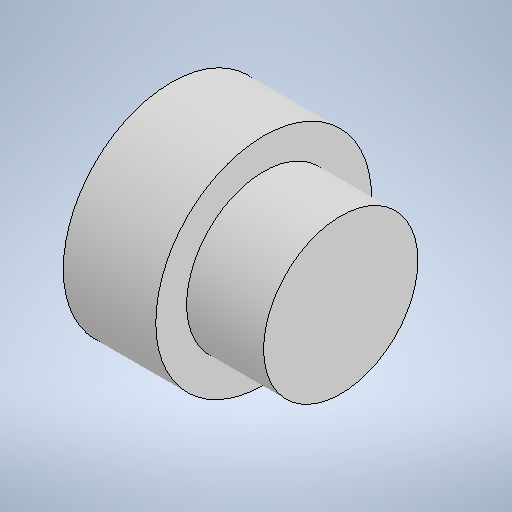
# Autodesk Inventor part: 1 part 16
Saved by Autodesk Inventor 2025 (Build 290162010, 162A)
## iProperties
Created: 2024-07-30
Part Number: 1 part 16
Material: Generic
Document SubType Name: Modeling
Designer: Fabri
Density: 1 g/cm^3
Appearance: Default
Author: Fabri
Autodesk Inventor part; units mm, degrees
ref_plane "YZ Plane" through (0, 0, 0) normal (1, 0, 0) x (0, 1, 0)
ref_plane "XZ Plane" through (0, 0, 0) normal (0, 1, 0) x (-1, 0, 0)
ref_plane "XY Plane" through (0, 0, 0) normal (0, 0, 1) x (1, 0, 0)
sketch "Sketch1" plane through (0, 0, 0) normal (0, 0, 1) x (1, 0, 0)
  line L0 (0, 0) -> (0, 7)
  line L1 (0, 7) -> (6, 7)
  line L2 (6, 7) -> (6, 5)
  line L3 (6, 5) -> (11, 5)
  line L4 (11, 5) -> (11, 0)
  line L5 (11, 0) -> (0, 0)
  dimension "d0" = 5
  dimension "d1" = 6
  dimension "d2" = 10
  dimension "d3" = 14
  constraints: 12 end point, 5 perpendicular, 1 vertical
  measures "d0" distance between parallel lines of L4 L2
  measures "d1" distance of L0.end L1.end
  measures "d2" diameter of L3 L5
  measures "d3" diameter of L1 L5
revolve "Revolution1" add sketch "Sketch1" angle 360 about axis through (11, 0, 0) along (-1, 0, 0)
sketch "Sketch2" plane through (0, 0, 0) normal (-1, 0, 0) x (0, 0, 1)
  circle A0 centre (0, 0) radius 7 projected
  point P0 (0, 0)
  constraints: 1 coincident
hole "Hole1" at (0, 0, 0) direction (1, 0, 0) diameter 4.134 depth 9 thread size "M5x0.8" class "6H" standard "ISO Metric profile"
body "Solid1"
